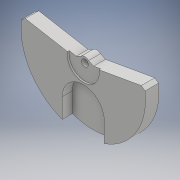
# Autodesk Inventor part: RescueKitThrow-Joint
Saved by Autodesk Inventor 2018.3 (Build 223284000, 284)
## iProperties
Created: 2019-02-13
Part Number: RescueKitThrow-Joint
Material: 一般
Document SubType Name: Modeling
Designer: TOMOKI
Density: 1 g/cm^3
Appearance: 既定
Author: TOMOKI
Autodesk Inventor part; units mm, degrees
ref_plane "YZ Plane" through (0, 0, 0) normal (1, 0, 0) x (0, 1, 0)
ref_plane "XZ Plane" through (0, 0, 0) normal (0, 1, 0) x (-1, 0, 0)
ref_plane "XY Plane" through (0, 0, 0) normal (0, 0, 1) x (1, 0, 0)
sketch "スケッチ1" plane through (0, 0, 0) normal (0, 1, 0) x (-1, 0, 0)
  arc A0 (54.0633, 37.5622) -> (47.6867, 37.5622) centre (50.875, 37) ccw
  circle A1 centre (50.875, 13.875) radius 12.5
  arc A2 (14.4371, 43.425) -> (87.3129, 43.425) centre (50.875, 37) ccw
  line L0 (50.875, 37) -> (87.3129, 43.425)
  line L1 (50.875, 37) -> (87.875, 37) construction
  line L2 (87.3129, 43.425) -> (50.875, 37)
  line L3 (50.875, 37) -> (14.4371, 43.425)
  point P0 (0, 0)
  dimension "d22" = 25
  dimension "d26" = 74
  dimension "d27" = 10
  constraints: 8 end point, 4 point on circle, 3 centre point, 2 point on line, 1 coincident, 1 collinear, 1 equal length, 1 horizontal
  measures "d22" diameter of A1
  measures "d26" diameter of A2
  measures "d27" angle of L1 L0
extrude "押し出し1" add sketch "スケッチ1" along normal blind 7
sketch "スケッチ2" plane through (0, 7, 0) normal (0, 1, 0) x (1, 0, 0)
  circle A0 centre (-50.875, -13.875) radius 12.5
  circle A1 centre (-50.875, -13.875) radius 12.5
  point P0 (0, 0)
  constraints: 2 centre point, 2 coincident, 1 concentric
extrude "押し出し2" add sketch "スケッチ2" against normal blind 2
sketch "スケッチ3" plane through (0, 0, 0) normal (0, -1, 0) x (1, 0, 0)
  circle A0 centre (-50.875, 13.875) radius 12.5 projected
  arc A1 (-47.6867, 37.5622) -> (-54.0633, 37.5622) centre (-50.875, 37) ccw projected
  circle A2 centre (-50.875, 13.875) radius 12.5 projected
  line L0 (-63.375, 13.875) -> (-38.375, 13.875)
  line L1 (-38.375, 13.875) -> (-38.375, 0)
  line L2 (-38.375, 0) -> (-63.375, 0)
  line L3 (-63.375, 0) -> (-63.375, 13.875)
  line L4 (-54.0633, 37.5622) -> (-87.3129, 43.425) projected
  arc A3 (-87.3129, 43.425) -> (-14.4371, 43.425) centre (-50.875, 37) ccw projected
  line L5 (-14.4371, 43.425) -> (-47.6867, 37.5622) projected
  point P0 (0, 0)
  constraints: 8 end point, 2 parallel, 1 horizontal, 1 horizontal alignment, 1 perpendicular, 1 other
extrude "押し出し3" cut sketch "スケッチ3" against normal blind 5 contours L1 A3 L3 A0 | A0 L0 | L1 L2 A3 | A3 L2 L3 picked at (-53.2419, 10.4459)
sketch "スケッチ4" plane through (0, 0, 0) normal (0, -1, 0) x (1, 0, 0)
  arc A0 (-47.6867, 37.5622) -> (-54.0633, 37.5622) centre (-50.875, 37) ccw projected
  circle A1 centre (-50.875, 37) radius 2.05
  arc A2 (-38.375, 13.875) -> (-63.375, 13.875) centre (-50.875, 13.875) ccw projected
  line L0 (-63.375, 2.1754) -> (-63.375, 13.875) projected
  line L1 (-38.375, 13.875) -> (-38.375, 2.1754) projected
  arc A3 (-38.375, 2.1754) -> (-14.4371, 43.425) centre (-50.875, 37) ccw projected
  line L2 (-14.4371, 43.425) -> (-47.6867, 37.5622) projected
  line L3 (-54.0633, 37.5622) -> (-87.3129, 43.425) projected
  arc A4 (-87.3129, 43.425) -> (-63.375, 2.1754) centre (-50.875, 37) ccw projected
  point P0 (0, 0)
  dimension "d12" = 4.1
  constraints: 1 centre point
  measures "d12" diameter of A1
extrude "押し出し4" cut sketch "スケッチ4" against normal blind 2.8 contours A1
sketch "スケッチ5" plane through (0, 7, 0) normal (0, 1, 0) x (1, 0, 0)
  arc A0 (-54.0633, -37.5622) -> (-47.6867, -37.5622) centre (-50.875, -37) ccw projected
  circle A1 centre (-50.875, -37) radius 1.25
  line L0 (-47.6867, -37.5622) -> (-14.4371, -43.425) projected
  arc A2 (-14.4371, -43.425) -> (-87.3129, -43.425) centre (-50.875, -37) ccw projected
  line L1 (-87.3129, -43.425) -> (-54.0633, -37.5622) projected
  point P0 (0, 0)
  dimension "d15" = 2.5
  constraints: 1 centre point, 1 coincident
  measures "d15" diameter of A1
extrude "押し出し5" cut sketch "スケッチ5" against normal blind 5 contours A1
chamfer "面取り1" distance 2 angle 45 4 edges at (-47.6867, 3.5, 37.5622) (-54.0633, 3.5, 37.5622) (-87.3129, 3.5, 43.425) (-14.4371, 3.5, 43.425)
sketch "スケッチ6" plane through (0, 0, 0) normal (0, -1, 0) x (1, 0, 0)
  circle A0 centre (-50.875, 37) radius 2.05 projected
  line L0 (-16.4067, 43.0777) -> (-14.1432, 41.4467) projected
  line L1 (-16.4067, 43.0777) -> (-45.7171, 37.9095) projected
  line L2 (-48.6254, 39.3282) -> (-45.7171, 37.9095) projected
  arc A1 (-48.6254, 39.3282) -> (-53.1246, 39.3282) centre (-50.875, 37) ccw projected
  line L3 (-56.0329, 37.9095) -> (-53.1246, 39.3282) projected
  line L4 (-56.0329, 37.9095) -> (-85.3433, 43.0777) projected
  line L5 (-87.6068, 41.4467) -> (-85.3433, 43.0777) projected
  arc A2 (-87.6068, 41.4467) -> (-63.375, 2.1754) centre (-50.875, 37) ccw projected
  line L6 (-63.375, 2.1754) -> (-63.375, 13.875) projected
  arc A3 (-38.375, 13.875) -> (-63.375, 13.875) centre (-50.875, 13.875) ccw projected
  line L7 (-38.375, 13.875) -> (-38.375, 2.1754) projected
  arc A4 (-38.375, 2.1754) -> (-14.1432, 41.4467) centre (-50.875, 37) ccw projected
  arc A5 (-60.2307, 38.6497) -> (-41.5193, 38.6497) centre (-50.875, 37) ccw
  circle A6 centre (-50.875, 37) radius 1.25 projected
  arc A7 (-87.6068, 41.4467) -> (-14.1432, 41.4467) centre (-50.875, 37) ccw
  point P0 (0, 0)
  dimension "d28" = 19
  constraints: 4 point on circle, 2 centre point, 2 coincident, 2 end point, 2 point on line
  measures "d28" diameter of A5
extrude "押し出し6" add sketch "スケッチ6" along normal blind 1 contours L0 A4 L7 A3 L6 A2 L5 L4 A5 L1
